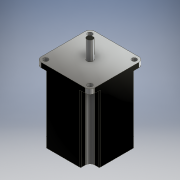
# Autodesk Inventor part: Stepper motor
Saved by Autodesk Inventor 2017 (Build 210142000, 142)
## iProperties
Created: 2017-09-06
Part Number: Stepper motor
Material: Generic
Document SubType Name: Modeling
Designer: Atef El-Naggar
Density: 1 g/cm^3
Appearance: Gunmetal
Author: Atef El-Naggar
Autodesk Inventor part; units mm, degrees
ref_plane "YZ Plane" through (0, 0, 0) normal (1, 0, 0) x (0, 1, 0)
ref_plane "XZ Plane" through (0, 0, 0) normal (0, 1, 0) x (-1, 0, 0)
ref_plane "XY Plane" through (0, 0, 0) normal (0, 0, 1) x (1, 0, 0)
sketch "Sketch1" plane through (0, 0, 0) normal (0, 0, 1) x (1, 0, 0)
  line L0 (17.5, 28.5) -> (-17.5, 28.5)
  line L1 (-28.5, 17.5) -> (-28.5, -17.5)
  line L2 (28.5, -17.5) -> (28.5, 17.5)
  arc A0 (-18.5, -23.5) -> (-23.5, -18.5) centre (-23.5, -23.5) ccw
  arc A1 (23.5, -18.5) -> (18.5, -23.5) centre (23.5, -23.5) ccw
  arc A2 (18.5, 23.5) -> (23.5, 18.5) centre (23.5, 23.5) ccw
  arc A3 (-23.5, 18.5) -> (-18.5, 23.5) centre (-23.5, 23.5) ccw
  line L3 (-23.5, 18.5) -> (-27.5, 18.5)
  line L4 (-18.5, 23.5) -> (-18.5, 27.5)
  line L5 (-23.5, -18.5) -> (-27.5, -18.5)
  line L6 (-18.5, -23.5) -> (-18.5, -27.5)
  line L7 (18.5, -23.5) -> (18.5, -27.5)
  line L8 (23.5, -18.5) -> (27.5, -18.5)
  line L9 (18.5, 23.5) -> (18.5, 27.5)
  line L10 (23.5, 18.5) -> (27.5, 18.5)
  line L11 (-17.5, -28.5) -> (17.5, -28.5)
  arc A4 (-28.5, -17.5) -> (-27.5, -18.5) centre (-27.5, -17.5) ccw
  arc A5 (17.5, -28.5) -> (18.5, -27.5) centre (17.5, -27.5) ccw
  arc A6 (-27.5, 18.5) -> (-28.5, 17.5) centre (-27.5, 17.5) ccw
  arc A7 (-17.5, 28.5) -> (-18.5, 27.5) centre (-17.5, 27.5) ccw
  arc A8 (-18.5, -27.5) -> (-17.5, -28.5) centre (-17.5, -27.5) ccw
  arc A9 (28.5, 17.5) -> (27.5, 18.5) centre (27.5, 17.5) ccw
  arc A10 (18.5, 27.5) -> (17.5, 28.5) centre (17.5, 27.5) ccw
  arc A11 (27.5, -18.5) -> (28.5, -17.5) centre (27.5, -17.5) ccw
  point P0 (0, 0)
  point P1 (18.5, 28.5)
  point P2 (-18.5, -28.5)
  point P3 (28.5, -18.5)
  point P4 (28.5, 18.5)
  dimension "d2" = 28.5
  dimension "d3" = 28.5
  dimension "d4" = 10
  dimension "d5" = 10
  dimension "d6" = 10
  dimension "d7" = 10
  dimension "d8" = 57
  dimension "d9" = 57
  dimension "d10" = 1
  constraints: 28 tangent, 24 end point, 24 point on circle, 16 point on line, 12 centre point, 7 equal radius, 5 perpendicular, 2 parallel, 1 horizontal
  measures "d2" distance from line of point (0, 0) L2
  measures "d3" distance from line of point (0, 0) L0
  measures "d4" diameter of A0
  measures "d5" diameter of A1
  measures "d6" diameter of A2
  measures "d7" diameter of A3
  measures "d8" distance between parallel lines of L11 L0
  measures "d9" distance between parallel lines of L1 L2
  measures "d10" radius of A4
extrude "Extrusion1" add sketch "Sketch1" along normal blind 15
sketch "Sketch2" plane through (0, 0, 15) normal (0, 0, 1) x (1, 0, 0)
  line L0 (17.5, 28.5) -> (-17.5, 28.5) projected
  arc A0 (-23.5, 18.5) -> (-18.5, 23.5) centre (-23.5, 23.5) ccw projected
  arc A1 (-23.5, 18.5) -> (-18.5, 23.5) centre (-23.5, 23.5) ccw projected
  line L1 (-23.5, 18.5) -> (-27.5, 18.5) projected
  arc A2 (-27.5, 18.5) -> (-28.5, 17.5) centre (-27.5, 17.5) ccw projected
  line L2 (-28.5, 17.5) -> (-28.5, -17.5) projected
  arc A3 (-28.5, -17.5) -> (-27.5, -18.5) centre (-27.5, -17.5) ccw projected
  line L3 (-27.5, -18.5) -> (-23.5, -18.5) projected
  arc A4 (-18.5, -23.5) -> (-23.5, -18.5) centre (-23.5, -23.5) ccw projected
  line L4 (-18.5, -23.5) -> (-18.5, -27.5) projected
  arc A5 (-18.5, -27.5) -> (-17.5, -28.5) centre (-17.5, -27.5) ccw projected
  line L5 (-17.5, -28.5) -> (17.5, -28.5) projected
  arc A6 (17.5, -28.5) -> (18.5, -27.5) centre (17.5, -27.5) ccw projected
  line L6 (18.5, -27.5) -> (18.5, -23.5) projected
  arc A7 (23.5, -18.5) -> (18.5, -23.5) centre (23.5, -23.5) ccw projected
  line L7 (23.5, -18.5) -> (27.5, -18.5) projected
  arc A8 (27.5, -18.5) -> (28.5, -17.5) centre (27.5, -17.5) ccw projected
  line L8 (28.5, -17.5) -> (28.5, 17.5) projected
  arc A9 (28.5, 17.5) -> (27.5, 18.5) centre (27.5, 17.5) ccw projected
  line L9 (27.5, 18.5) -> (23.5, 18.5) projected
  arc A10 (18.5, 23.5) -> (23.5, 18.5) centre (23.5, 23.5) ccw projected
  line L10 (18.5, 23.5) -> (18.5, 27.5) projected
  arc A11 (18.5, 27.5) -> (17.5, 28.5) centre (17.5, 27.5) ccw projected
  line L11 (17.5, 28.5) -> (-17.5, 28.5) projected
  arc A12 (-17.5, 28.5) -> (-18.5, 27.5) centre (-17.5, 27.5) ccw projected
  line L12 (-18.5, 27.5) -> (-18.5, 23.5) projected
  point P0 (0, 0)
extrude "Extrusion2" add sketch "Sketch2" along normal blind 46
sketch "Sketch3" plane through (0, 0, 61) normal (0, 0, 1) x (1, 0, 0)
  arc A0 (-23.5, 18.5) -> (-18.5, 23.5) centre (-23.5, 23.5) ccw projected
  line L0 (-23.5, 18.5) -> (-27.5, 18.5) projected
  arc A1 (-27.5, 18.5) -> (-28.5, 17.5) centre (-27.5, 17.5) ccw projected
  line L1 (-28.5, 17.5) -> (-28.5, -17.5) projected
  arc A2 (-28.5, -17.5) -> (-27.5, -18.5) centre (-27.5, -17.5) ccw projected
  line L2 (-27.5, -18.5) -> (-23.5, -18.5) projected
  arc A3 (-18.5, -23.5) -> (-23.5, -18.5) centre (-23.5, -23.5) ccw projected
  line L3 (-18.5, -23.5) -> (-18.5, -27.5) projected
  arc A4 (-18.5, -27.5) -> (-17.5, -28.5) centre (-17.5, -27.5) ccw projected
  line L4 (-17.5, -28.5) -> (17.5, -28.5) projected
  arc A5 (17.5, -28.5) -> (18.5, -27.5) centre (17.5, -27.5) ccw projected
  line L5 (18.5, -27.5) -> (18.5, -23.5) projected
  arc A6 (23.5, -18.5) -> (18.5, -23.5) centre (23.5, -23.5) ccw projected
  line L6 (23.5, -18.5) -> (27.5, -18.5) projected
  arc A7 (27.5, -18.5) -> (28.5, -17.5) centre (27.5, -17.5) ccw projected
  line L7 (28.5, -17.5) -> (28.5, 17.5) projected
  arc A8 (28.5, 17.5) -> (27.5, 18.5) centre (27.5, 17.5) ccw projected
  line L8 (27.5, 18.5) -> (23.5, 18.5) projected
  arc A9 (18.5, 23.5) -> (23.5, 18.5) centre (23.5, 23.5) ccw projected
  line L9 (18.5, 23.5) -> (18.5, 27.5) projected
  arc A10 (18.5, 27.5) -> (17.5, 28.5) centre (17.5, 27.5) ccw projected
  line L10 (17.5, 28.5) -> (-17.5, 28.5) projected
  arc A11 (-17.5, 28.5) -> (-18.5, 27.5) centre (-17.5, 27.5) ccw projected
  line L11 (-18.5, 27.5) -> (-18.5, 23.5) projected
  point P0 (0, 0)
extrude "Extrusion3" add sketch "Sketch3" along normal blind 10
sketch "Sketch4" plane through (0, 0, 71) normal (0, 0, 1) x (1, 0, 0)
  line L0 (-23.5, -28.5) -> (23.5, -28.5)
  line L1 (28.5, -23.5) -> (28.5, 23.5)
  line L2 (23.5, 28.5) -> (-23.5, 28.5)
  line L3 (-28.5, 23.5) -> (-28.5, -23.5)
  line L4 (-27.0355, -27.0355) -> (28.5, 28.5) construction
  line L5 (28.5, -28.5) -> (-28.5, 28.5) construction
  arc A0 (-23.5, 28.5) -> (-28.5, 23.5) centre (-23.5, 23.5) ccw
  arc A1 (28.5, 23.5) -> (23.5, 28.5) centre (23.5, 23.5) ccw
  arc A2 (23.5, -28.5) -> (28.5, -23.5) centre (23.5, -23.5) ccw
  arc A3 (-28.5, -23.5) -> (-23.5, -28.5) centre (-23.5, -23.5) ccw
  line L6 (17.5, 28.5) -> (-17.5, 28.5) projected
  circle A4 centre (-23.5, 23.5) radius 2.5
  circle A5 centre (23.5, 23.5) radius 2.5
  circle A6 centre (23.5, -23.5) radius 2.5
  circle A7 centre (-23.5, -23.5) radius 2.5
  point P0 (0, 0)
  dimension "d17" = 57
  dimension "d18" = 10
  dimension "d19" = 10
  dimension "d20" = 10
  dimension "d21" = 10
  dimension "d22" = 28.5
  dimension "d23" = 5
  dimension "d24" = 5
  dimension "d25" = 5
  dimension "d26" = 5
  constraints: 12 end point, 9 point on circle, 8 centre point, 8 tangent, 4 coincident, 2 parallel, 1 horizontal, 1 midpoint, 1 perpendicular, 1 point on line
  measures "d17" distance of L5.end L4.end
  measures "d18" diameter of A0
  measures "d19" diameter of A1
  measures "d20" diameter of A2
  measures "d21" diameter of A3
  measures "d22" distance from line of point (0, 0) L2
  measures "d23" diameter of A4
  measures "d24" diameter of A5
  measures "d25" diameter of A6
  measures "d26" diameter of A7
extrude "Extrusion4" add sketch "Sketch4" along normal blind 5
sketch "Sketch5" plane through (0, 0, 76) normal (0, 0, 1) x (1, 0, 0)
  circle A0 centre (0, 0) radius 3.15
  dimension "d29" = 6.3
  constraints: 1 centre point, 1 coincident
  measures "d29" diameter of A0
extrude "Extrusion5" add sketch "Sketch5" along normal blind 20
sketch "Sketch6" plane through (0, 0, 96) normal (0, 0, 1) x (1, 0, 0)
  arc A0 (1.7029, 2.65) -> (-1.7029, 2.65) centre (0, 0) ccw
  line L0 (1.7029, 2.65) -> (-1.7029, 2.65)
  circle A1 centre (0, 0) radius 3.15 projected
  arc A2 (1.7029, 2.65) -> (-1.7029, 2.65) centre (0, 0) ccw
  constraints: 4 point on circle, 2 centre point, 2 end point, 1 coincident, 1 horizontal
extrude "Extrusion6" cut sketch "Sketch6" against normal blind 16 contours L0 A0
body "Solid1"
